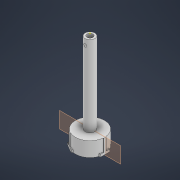
# Autodesk Inventor part: kneading shaft
Saved by Autodesk Inventor 2021 (Build 250183000, 183)
## iProperties
Created: 2022-05-20
Part Number: kneading shaft
Material: Generic
Document SubType Name: Modeling
Designer: techv
Density: 1 g/cm^3
Appearance: Default
Author: techv
Autodesk Inventor part; units mm, degrees
ref_plane "YZ Plane" through (0, 0, 0) normal (1, 0, 0) x (0, 1, 0)
ref_plane "XZ Plane" through (0, 0, 0) normal (0, 1, 0) x (-1, 0, 0)
ref_plane "XY Plane" through (0, 0, 0) normal (0, 0, 1) x (1, 0, 0)
sketch "Sketch1" plane through (0, 0, 0) normal (0, 1, 0) x (-1, 0, 0)
  circle A0 centre (0, 0) radius 5
  dimension "d0" = 10
  constraints: 1 centre point, 1 coincident
  measures "d0" diameter of A0
extrude "Extrusion1" add sketch "Sketch1" along normal blind 100
sketch "Sketch2" plane through (0, 0, 0) normal (0, -1, 0) x (1, 0, 0)
  circle A0 centre (0, 0) radius 15
  dimension "d3" = 30
  constraints: 1 centre point, 1 coincident
  measures "d3" diameter of A0
extrude "Extrusion2" add sketch "Sketch2" against normal blind 15
sketch "Sketch3" plane through (0, 0, 0) normal (0, -1, 0) x (1, 0, 0)
  line L0 (13.75, -5) -> (16.25, -5)
  line L1 (16.25, -5) -> (16.25, 5)
  line L2 (16.25, 5) -> (13.75, 5)
  line L3 (13.75, 5) -> (13.75, -5)
  circle A0 centre (0, 0) radius 15 projected
  line L4 (13.75, -5) -> (16.25, 5) construction
  line L5 (16.25, -5) -> (13.75, 5) construction
  point P0 (15, 0)
  point P1 (14.25, 4.6837)
  point P2 (14.25, -4.6837)
  point P3 (14.1421, 5)
  point P4 (14.1421, -5)
  dimension "d6" = 2.5
  dimension "d7" = 10
  constraints: 12 end point, 2 midpoint, 2 parallel, 1 horizontal, 1 perpendicular, 2 other
  measures "d6" distance of L2.end L1.end
  measures "d7" distance of L1.end L0.end
extrude "Extrusion3" add sketch "Sketch3" against normal blind 2.5 contours A0 L2 L1 L0
sketch "Sketch4" plane through (0, 2.5, 0) normal (0, 1, 0) x (1, 0, 0)
  circle A0 centre (0, 0) radius 15 projected
  circle A1 centre (0, 0) radius 5 projected
  line L0 (16.25, -5) -> (16.25, 5) projected
  line L1 (13.75, 1.25) -> (16.25, 1.25)
  line L2 (16.25, 1.25) -> (16.25, -1.25)
  line L3 (16.25, -1.25) -> (13.75, -1.25)
  line L4 (13.75, -1.25) -> (13.75, 1.25)
  circle A2 centre (0, 0) radius 15 projected
  line L5 (13.75, 1.25) -> (16.25, -1.25) construction
  line L6 (16.25, 1.25) -> (13.75, -1.25) construction
  point P0 (15, 0)
  point P1 (14.9478, -1.25)
  point P2 (14.9478, 1.25)
  dimension "d10" = 2.5
  constraints: 12 end point, 2 midpoint, 2 parallel, 1 horizontal, 1 horizontal alignment, 1 perpendicular, 1 point on line, 1 other
  measures "d10" distance of L1.end L2.end
extrude "Extrusion4" add sketch "Sketch4" along normal up to surface (12.5 mm away) contours A0 L1 L0 L3
sketch "Sketch5" plane through (16.25, 0, 5) normal (1, 0, 0) x (0, 0, -1)
  line L0 (10, 0) -> (0, 0) projected
  line L1 (10, 0) -> (10, 2.5) projected
  line L2 (6.25, 2.5) -> (10, 2.5) projected
  line L3 (6.25, 2.5) -> (6.25, 15) projected
  line L4 (3.75, 15) -> (6.25, 15) projected
  line L5 (3.75, 2.5) -> (3.75, 15) projected
  line L6 (0, 2.5) -> (3.75, 2.5) projected
  line L7 (0, 0) -> (0, 2.5) projected
  point P0 (5, 0)
extrude "Extrusion5" cut sketch "Sketch5" against normal blind 0.7
pattern_circular "Circular Pattern1" count 3 over 360 about axis through (0, 0, 0) along (0, 1, 0) of "Extrusion4", "Extrusion3", "Extrusion5"
sketch "Sketch6" plane through (0, 100, 0) normal (0, 1, 0) x (1, 0, 0)
  point P0 (0, 0)
sketch "Sketch7" plane through (0, 100, 0) normal (0, 1, 0) x (1, 0, 0)
  circle A0 centre (0, 0) radius 5 projected
extrude "Extrusion6" cut sketch "Sketch7" against normal blind 2
sketch "Sketch8" plane through (0, 98, 0) normal (0, 1, 0) x (1, 0, 0)
  circle A0 centre (0, 0) radius 3
  dimension "d20" = 6
  constraints: 1 centre point, 1 coincident
  measures "d20" diameter of A0
extrude "Extrusion7" cut sketch "Sketch8" against normal blind 14
ref_plane "Work Plane1" through (0, 15, 0) normal (0, 0, 1) x (1, 0, 0)
sketch "Sketch9" plane through (0, 15, 0) normal (0, 0, 1) x (1, 0, 0)
  line L0 (-3, 69) -> (3, 69) projected
  line L1 (-3, 83) -> (-3, 69) projected
  line L2 (3, 83) -> (3, 69) projected
  line L3 (-5, 83) -> (5, 83) projected
  circle A0 centre (0, 77) radius 1.5
  line L4 (0, 69) -> (0, 83)
  point P0 (0, -15)
  dimension "d23" = 3
  dimension "d24" = 0
  dimension "d25" = 8
  constraints: 2 end point, 2 midpoint, 1 centre point
  measures "d23" diameter of A0
  measures "d24" distance from line of L4 A0.centre
  measures "d25" distance from line of L0 A0.centre
extrude "Extrusion8" cut sketch "Sketch9" against normal mid plane 10 contours L4 A0 | A0 L4
sketch "Sketch10" plane through (0, 98, 0) normal (0, 1, 0) x (1, 0, 0)
  circle A0 centre (0, 0) radius 3 projected
  circle A1 centre (0, 0) radius 5 projected
extrude "Extrusion9" add sketch "Sketch10" along normal blind 5
sketch "Sketch11" plane through (0, 103, 0) normal (0, 1, 0) x (1, 0, 0)
  circle A0 centre (0, 0) radius 5 projected
  circle A1 centre (0, 0) radius 3 projected
extrude "Extrusion10" cut sketch "Sketch11" against normal blind 5
body "Solid1"
